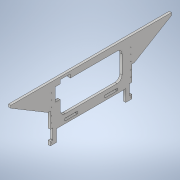
# Autodesk Inventor part: open_case
Saved by Autodesk Inventor 2020 (Build 240168000, 168)
## iProperties
Created: 2019-12-18
Part Number: open_case
Material: Generic
Document SubType Name: Modeling
Designer: fabfarm
Density: 1 g/cm^3
Appearance: Default
Author: fabfarm
Autodesk Inventor part; units mm, degrees
ref_plane "YZ Plane" through (0, 0, 0) normal (1, 0, 0) x (0, 1, 0)
ref_plane "XZ Plane" through (0, 0, 0) normal (0, 1, 0) x (-1, 0, 0)
ref_plane "XY Plane" through (0, 0, 0) normal (0, 0, 1) x (1, 0, 0)
sketch "Sketch1" plane through (0, 0, 0) normal (1, 0, 0) x (0, 1, 0)
  line L0 (-163.975, -330) -> (163.975, -330)
  line L1 (163.975, -330) -> (163.975, 330)
  line L2 (163.975, 330) -> (-163.975, 330)
  line L3 (-163.975, 330) -> (-163.975, -330)
  line L4 (-163.975, -330) -> (163.975, 330) construction
  line L5 (163.975, -330) -> (-163.975, 330) construction
  point P0 (0, 0)
  dimension "d0" = 660
  dimension "d1" = 327.95
  constraints: 12 end point, 2 midpoint, 2 parallel, 1 horizontal, 1 perpendicular
  measures "d0" distance of L0.end L1.end
  measures "d1" distance of L0.start L0.end
extrude "Extrusion1" add sketch "Sketch1" along normal blind 18.55
sketch "Sketch2" plane through (18.55, 0, 0) normal (1, 0, 0) x (0, 0, -1)
  line L0 (-330, 163.975) -> (-330, -163.975) projected
  line L1 (-330, 60.925) -> (-311.45, 60.925)
  line L2 (-311.45, 60.925) -> (-311.45, -39.275)
  line L3 (-311.45, -39.275) -> (-330, -39.275)
  line L4 (-330, -39.275) -> (-330, 60.925)
  line L5 (330, 163.975) -> (-330, 163.975) projected
  line L6 (-330, -163.975) -> (330, -163.975) projected
  point P0 (-330, 163.875)
  point P1 (-330, -163.875)
  point P2 (330, 163.875)
  point P3 (330, -163.875)
  point P4 (330, -163.975)
  dimension "d20" = 100.2
  dimension "d21" = 103.05
  dimension "d22" = 124.7
  dimension "d23" = 18.55
  constraints: 8 end point, 2 parallel, 1 horizontal, 1 perpendicular, 1 point on line, 2 other
  measures "d20" distance of L1.end L2.end
  measures "d23" distance of L1.start L1.end
extrude "Extrusion2" [suppressed]
mirror "Mirror1" [suppressed]
sketch "Sketch3" plane through (18.55, 0, 0) normal (1, 0, 0) x (0, 0, -1)
  line L0 (210, -113.975) -> (-210, -113.975)
  line L1 (-250, -73.975) -> (-250, 73.975)
  line L2 (-210, 113.975) -> (210, 113.975)
  line L3 (250, 73.975) -> (250, -73.975)
  line L4 (250, -113.975) -> (-250, 113.975) construction
  line L5 (-250, -113.975) -> (250, 113.975) construction
  arc A0 (-210, 113.975) -> (-250, 73.975) centre (-210, 73.975) ccw
  arc A1 (-250, -73.975) -> (-210, -113.975) centre (-210, -73.975) ccw
  arc A2 (250, 73.975) -> (210, 113.975) centre (210, 73.975) ccw
  arc A3 (210, -113.975) -> (250, -73.975) centre (210, -73.975) ccw
  line L6 (-330, 163.975) -> (-330, -163.975) projected
  line L7 (330, 163.975) -> (-330, 163.975) projected
  point P0 (0, 0)
  point P1 (-330, -39.175)
  point P2 (-330, -163.875)
  point P3 (330, 163.875)
  point P4 (-330, 163.875)
  dimension "d17" = 40
  dimension "d40" = 80
  dimension "d41" = 50
  constraints: 12 end point, 8 point on circle, 8 point on line, 8 tangent, 4 centre point, 3 equal radius, 2 midpoint, 2 parallel, 1 horizontal, 1 perpendicular, 1 other
  measures "d17" radius of A0
  measures "d40" distance between parallel lines of L6 L1
extrude "Extrusion3" cut sketch "Sketch3" against normal blind 18.55
sketch "Esquisse4" plane through (18.55, 0, 0) normal (1, 0, 0) x (0, 0, -1)
  circle A0 centre (-312.5725, 59.9025) radius 1.5875
  circle A1 centre (-312.5725, -38.0525) radius 1.5875
  line L0 (-312.5725, 59.9025) -> (-311.45, 61.025) construction
  line L1 (-311.45, 61.025) -> (-311.45, -39.175) projected
  line L2 (210, 113.975) -> (-210, 113.975) projected
  line L3 (0, 113.975) -> (0, -113.975) construction
  line L4 (-210, -113.975) -> (210, -113.975) projected
  circle A2 centre (312.5725, 59.9025) radius 1.5875
  circle A3 centre (312.5725, -38.0525) radius 1.5875
  line L5 (312.5725, 59.9025) -> (311.45, 61.025) construction
  point P0 (0, 0)
  point P1 (311.45, 61.025)
  point P2 (311.45, -39.175)
  point P3 (311.45, -39.175)
  dimension "d24" = 3.175
  dimension "d39" = 45
  constraints: 6 end point, 4 symmetric about line, 2 midpoint, 2 vertical, 1 vertical alignment, 12 other
  measures "d39" angle of L1 L0
extrude "Extrusion4" [suppressed]
sketch "Esquisse5" plane through (18.55, 0, 0) normal (1, 0, 0) x (0, 0, -1)
  line L0 (-211.5, -163.975) -> (-111.4, -163.975)
  line L1 (-111.4, -163.975) -> (-111.4, -145.325)
  line L2 (-111.4, -145.325) -> (-211.5, -145.325)
  line L3 (-211.5, -145.325) -> (-211.5, -163.975)
  line L4 (111.4, -163.975) -> (211.5, -163.975)
  line L5 (211.5, -163.975) -> (211.5, -145.325)
  line L6 (211.5, -145.325) -> (111.4, -145.325)
  line L7 (111.4, -145.325) -> (111.4, -163.975)
  line L8 (-330, 163.975) -> (-330, -163.975) projected
  line L9 (330, -163.975) -> (330, 163.975) projected
  line L10 (210, -113.975) -> (-210, -113.975) projected
  line L11 (-330, -163.975) -> (330, -163.975) projected
  point P0 (0, 0)
  point P1 (-330, -163.875)
  point P2 (330, -163.875)
  point P3 (-330, -39.175)
  point P4 (330, -39.175)
  point P5 (330, 61.025)
  dimension "d27" = 100.1
  dimension "d28" = 100.1
  dimension "d29" = 118.5
  dimension "d30" = 118.5
  dimension "d38" = 18.65
  constraints: 16 end point, 4 parallel, 3 horizontal, 2 perpendicular, 1 collinear, 1 point on line, 1 other
  measures "d27" distance of L1.end L2.end
  measures "d28" distance of L5.end L6.end
  measures "d29" distance between parallel lines of L8 L3
  measures "d30" distance between parallel lines of L9 L5
  measures "d38" distance of L0.end L1.end
extrude "Extrusion5" cut sketch "Esquisse5" against normal blind 20
sketch "Esquisse6" plane through (18.55, 0, 0) normal (1, 0, 0) x (0, 0, -1)
  circle A0 centre (-210.3686, -146.4564) radius 1.6
  circle A1 centre (-112.5314, -146.4564) radius 1.6
  line L0 (-211.5, -163.975) -> (-211.5, -145.325) projected
  line L1 (-211.5, -145.325) -> (-210.3686, -146.4564) construction
  circle A2 centre (112.5314, -146.4564) radius 1.6
  circle A3 centre (210.3686, -146.4564) radius 1.6
  point P0 (0, 0)
  point P1 (-111.4, -145.325)
  point P2 (111.4, -145.325)
  point P3 (211.5, -145.325)
  dimension "d42" = 3.2
  dimension "d43" = 45
  constraints: 3 horizontal alignment, 2 end point, 12 other
  measures "d43" angle of L0 L1
extrude "Extrusion6" cut sketch "Esquisse6" against normal blind 20
sketch "Esquisse8" plane through (18.55, 0, 0) normal (1, 0, 0) x (0, 0, -1)
  line L0 (330, -163.975) -> (330, -181.7314)
  line L1 (280, -183.975) -> (-280, -183.975)
  line L2 (-330, -183.875) -> (-330, -163.975)
  line L3 (330, -163.975) -> (330, 163.975) projected
  line L4 (-280, -183.975) -> (-280, -280.425)
  line L5 (-280, -280.425) -> (-330, -280.425)
  line L6 (-330, -280.425) -> (-330, -183.875)
  line L7 (280, -183.975) -> (280, -280.425)
  line L8 (280, -280.425) -> (330, -280.425)
  line L9 (330, -280.425) -> (330, -181.7314)
  line L10 (-330, -163.975) -> (-211.5, -163.975) projected
  line L11 (-111.4, -163.975) -> (-111.4, -164.175)
  line L12 (-111.4, -164.175) -> (-211.5, -164.175)
  line L13 (-211.5, -164.175) -> (-211.5, -163.975)
  line L14 (-111.4, -147.5877) -> (-111.4, -163.975) projected
  line L15 (-111.4, -163.975) -> (111.4, -163.975) projected
  line L16 (-330, -163.975) -> (-211.5, -163.975)
  line L17 (111.4, -163.975) -> (111.4, -147.5877) projected
  line L18 (211.5, -163.975) -> (211.5, -164.175)
  line L19 (211.5, -164.175) -> (111.4, -164.175)
  line L20 (111.4, -164.175) -> (111.4, -163.975)
  line L21 (211.5, -147.5877) -> (211.5, -163.975) projected
  line L22 (-111.4, -163.975) -> (111.4, -163.975)
  line L23 (211.5, -163.975) -> (330, -163.975)
  point P0 (0, 0)
  point P1 (330, -39.175)
  point P2 (330, 61.025)
  dimension "d47" = 50
  dimension "d77" = 0.2
  dimension "d78" = 20
  dimension "d80" = 116.45
  constraints: 37 end point, 8 collinear, 7 parallel, 3 horizontal, 2 perpendicular, 2 point on line, 2 vertical
  measures "d47" distance of L4.end L5.end
  measures "d77" distance between parallel lines of L15 L12
  measures "d78" distance between parallel lines of L1 L23
  measures "d80" distance between parallel lines of L8 L23
extrude "Extrusion7" add sketch "Esquisse8" against normal blind 18.55
sketch "Esquisse9" plane through (18.55, 0, 0) normal (1, 0, 0) x (0, 0, -1)
  line L0 (-330, -248.975) -> (-311.35, -248.975)
  line L1 (-311.35, -248.975) -> (-311.35, -163.775)
  line L2 (-311.35, -163.775) -> (-330, -163.775)
  line L3 (-330, -163.775) -> (-330, -248.975)
  line L4 (330, -248.975) -> (311.35, -248.975)
  line L5 (311.35, -248.975) -> (311.35, -163.775)
  line L6 (311.35, -163.775) -> (330, -163.775)
  line L7 (330, -163.775) -> (330, -248.975)
  line L8 (330, -280.425) -> (330, 163.975) projected
  line L9 (-330, 163.975) -> (-330, -280.425) projected
  line L10 (-330, -280.425) -> (-280, -280.425) projected
  point P0 (0, 0)
  point P1 (330, -39.175)
  point P2 (-330, -39.175)
  point P3 (330, -163.975)
  point P4 (-330, -163.975)
  dimension "d50" = 85.2
  dimension "d51" = 31.45
  dimension "d52" = 18.65
  constraints: 16 end point, 5 collinear, 4 parallel, 2 horizontal, 2 perpendicular
  measures "d50" distance of L4.end L5.end
  measures "d51" distance between parallel lines of L10 L0
  measures "d52" distance of L0.start L0.end
extrude "Extrusion8" cut sketch "Esquisse9" against normal blind 18.55
sketch "Esquisse10" plane through (18.55, 0, 0) normal (1, 0, 0) x (0, 0, -1)
  line L0 (-330, -36.025) -> (-350, -36.025)
  line L1 (-650, 163.975) -> (-330, 163.975)
  line L2 (-650, 163.975) -> (-650, 143.975)
  line L3 (-650, 143.975) -> (-350, -36.025)
  line L4 (330, 163.975) -> (-330, 163.975) projected
  line L5 (0, 163.975) -> (0, -183.975) construction
  line L6 (-280, -183.975) -> (280, -183.975) projected
  line L7 (-330, 163.975) -> (-330, -36.025)
  line L8 (-330, 163.975) -> (-330, -163.775) projected
  line L9 (330, -36.025) -> (350, -36.025)
  line L10 (650, 163.975) -> (329.9999, 163.975)
  line L11 (650, 163.975) -> (650, 143.975)
  line L12 (650, 143.975) -> (350, -36.025)
  line L13 (329.9999, 163.975) -> (330, -36.025)
  point P0 (0, 0)
  dimension "d56" = 20
  dimension "d59" = 320
  dimension "d67" = 200
  dimension "d68" = 20
  constraints: 22 end point, 4 symmetric about line, 3 collinear, 2 midpoint, 1 horizontal, 1 parallel, 1 vertical
  measures "d56" distance of L1.start L2.end
  measures "d59" distance of L1.start L1.end
  measures "d67" distance of L1.end L0.start
  measures "d68" distance of L0.start L0.end
extrude "Extrusion9" add sketch "Esquisse10" against normal blind 18.55
sketch "Esquisse11" plane through (18.55, 0, 0) normal (1, 0, 0) x (0, 0, -1)
  circle A0 centre (-320.725, 35.925) radius 2.25
  circle A1 centre (-320.725, -14.075) radius 2.25
  line L0 (330, 164.075) -> (-330, 164.075) projected
  line L1 (0, 164.075) -> (0, -183.975) construction
  line L2 (-280, -183.975) -> (280, -183.975) projected
  line L3 (330, 61.025) -> (311.45, 61.025)
  line L4 (320.725, 61.025) -> (320.725, -39.175) construction
  line L5 (311.45, -39.175) -> (330, -39.175)
  circle A2 centre (320.725, 35.925) radius 2.25
  circle A3 centre (320.725, -14.075) radius 2.25
  line L6 (-330, -36.025) -> (-330, -163.775) projected
  line L7 (-350, -36.025) -> (-330, -36.025) projected
  circle A4 centre (-320.725, -74.075) radius 2.25
  circle A5 centre (-320.725, -124.075) radius 2.25
  circle A6 centre (320.725, -74.075) radius 2.25
  circle A7 centre (320.725, -124.075) radius 2.25
  circle A8 centre (-320.725, 85.925) radius 2.25
  circle A9 centre (-320.725, 135.925) radius 2.25
  circle A10 centre (320.725, 85.925) radius 2.25
  circle A11 centre (320.725, 135.925) radius 2.25
  point P0 (0, 0)
  dimension "d62" = 50
  dimension "d64" = 4.5
  dimension "d81" = 9.275
  dimension "d82" = 21.95
  dimension "d90" = 60
  dimension "d91" = 50
  dimension "d103" = 50
  dimension "d104" = 50
  constraints: 12 centre point, 8 end point, 6 symmetric about line, 5 equal radius, 5 vertical alignment, 2 midpoint, 2 point on line, 6 other
  measures "d62" distance of A1.centre A0.centre
  measures "d64" diameter of A0
  measures "d81" distance from line of L6 A1.centre
  measures "d82" distance from line of A1.centre L7
  measures "d90" distance of A4.centre A1.centre
  measures "d91" distance of A5.centre A4.centre
  measures "d103" distance of A8.centre A0.centre
  measures "d104" distance of A9.centre A8.centre
extrude "Extrusion10" cut sketch "Esquisse11" against normal blind 18.55 contours A0 | A1 | A2 | A3 | A4 | A5 | A6 | A7 | A8 | A10
sketch "Esquisse12" plane through (18.55, 0, 0) normal (1, 0, 0) x (0, 0, -1)
  line L0 (-311.35, -163.775) -> (-311.35, -248.975) projected
  circle A0 centre (-312.4814, -164.9064) radius 1.6
  circle A1 centre (-312.4814, -247.8436) radius 1.6
  line L1 (-311.35, -248.975) -> (-312.4814, -247.8436)
  line L2 (-311.35, -248.975) -> (-330, -248.975) projected
  line L3 (210, -113.975) -> (-210, -113.975) projected
  line L4 (0, -113.975) -> (0, -183.975) construction
  line L5 (-280, -183.975) -> (280, -183.975) projected
  circle A2 centre (312.4814, -164.9064) radius 1.6
  circle A3 centre (312.4814, -247.8436) radius 1.6
  line L6 (311.35, -248.975) -> (312.4814, -247.8436)
  line L7 (311.35, -248.975) -> (330, -248.975)
  circle A4 centre (-210.3686, -163.0436) radius 1.6
  circle A5 centre (-112.5314, -163.0436) radius 1.6
  line L8 (-211.5, -164.175) -> (-210.3686, -163.0436) construction
  circle A6 centre (210.3686, -163.0436) radius 1.6
  circle A7 centre (112.5314, -163.0436) radius 1.6
  line L9 (211.5, -164.175) -> (210.3686, -163.0436) construction
  line L10 (-111.4, -164.175) -> (-211.5, -164.175) projected
  point P0 (0, 0)
  point P1 (-311.35, -163.975)
  dimension "d70" = 3.2
  dimension "d74" = 3.2
  dimension "d69" = 45
  dimension "d83" = 45
  constraints: 12 end point, 7 symmetric about line, 2 centre point, 2 midpoint, 2 vertical, 1 coincident, 1 horizontal alignment, 1 vertical alignment, 20 other
  measures "d69" angle of L2 L1
  measures "d83" angle of L10 L8
extrude "Extrusion11" cut sketch "Esquisse12" against normal blind 18.55
sketch "Esquisse13" plane through (18.55, 0, 0) normal (1, 0, 0) x (0, 0, -1)
  line L0 (250, 73.975) -> (250, -73.975) projected
  line L1 (-290, 113.975) -> (-210, 113.975)
  line L2 (-210, 113.975) -> (-210, 6.025)
  line L3 (-210, 6.025) -> (-290, 6.025)
  line L4 (-290, 6.025) -> (-290, 113.975)
  line L5 (-250, -73.975) -> (-250, 73.975) projected
  point P0 (0, 0)
  dimension "d85" = 80
  dimension "d89" = 40
  constraints: 8 end point, 2 parallel, 1 coincident, 1 horizontal, 1 perpendicular
  measures "d85" distance from line of L0.end L3
  measures "d89" distance between parallel lines of L5 L4
extrude "Extrusion12" cut sketch "Esquisse13" against normal blind 18.55
fillet "Congé1" radius 2 3 edges at (9.275, 113.975, 290) (9.275, 6.025, 290) (9.275, 6.025, 250)
sketch "Esquisse14" plane through (18.55, 0, 0) normal (1, 0, 0) x (0, 0, -1)
  circle A0 centre (-321, -263.975) radius 2.25
  line L0 (-330, -36.025) -> (-330, -163.775) projected
  line L1 (-313.6127, -248.975) -> (-330, -248.975) projected
  circle A1 centre (321, -263.975) radius 2.25
  line L2 (330, -163.775) -> (330, -36.025) projected
  point P0 (0, 0)
  point P1 (-330, -280.425)
  point P2 (330, -280.425)
  point P3 (330, -248.975)
  dimension "d92" = 9
  dimension "d93" = 15
  dimension "d94" = 4.5
  dimension "d95" = 9
  constraints: 2 centre point, 1 equal radius, 1 horizontal alignment
  measures "d92" distance from line of A0.centre L0
  measures "d93" distance from line of L1 A0.centre
  measures "d94" diameter of A0
  measures "d95" distance from line of L2 A1.centre
extrude "Extrusion13" cut sketch "Esquisse14" against normal blind 18.55
sketch "Esquisse15" plane through (0, 0, 0) normal (-1, 0, 0) x (0, 0, 1)
  line L0 (-210, 113.975) -> (288, 113.975) projected
  line L1 (250, 113.975) -> (170, 113.975)
  line L2 (170, 113.975) -> (170, 143.975)
  line L3 (170, 143.975) -> (250, 143.975)
  line L4 (250, 143.975) -> (250, 113.975)
  line L5 (250, 4.025) -> (250, -73.975) projected
  point P0 (0, 0)
  point P1 (170, 113.975)
  dimension "d98" = 80
  dimension "d99" = 30
  constraints: 8 end point, 2 parallel, 1 collinear, 1 horizontal, 1 perpendicular, 1 point on line
  measures "d98" distance of L2.end L3.end
  measures "d99" distance of L1.end L2.end
extrude "Extrusion14" cut sketch "Esquisse15" against normal blind 18.55
fillet "Congé2" radius 2 4 edges at (9.275, 143.975, 250) (9.275, 113.975, 250) (9.275, 143.975, 170) (9.275, 113.975, 170)
body "Solid1"
